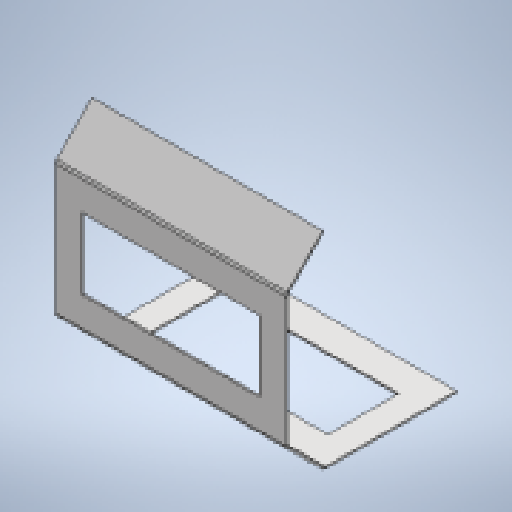
# Autodesk Inventor part: ANP 1454 BOTTOM DS box wall 1
Saved by Autodesk Inventor 2025 (Build 290162010, 162A)
## iProperties
Created: 2024-12-09
Part Number: ANP 1454 BOTTOM DS box wall 1
Material: Stainless Steel
Document SubType Name: Sheet Metal
Designer: user
Mass: 3269.02 g
Surface Area: 1007.63 cm^2
Volume: 408.627 cm^3
Density: 8 g/cm^3
Flat Pattern Width: 41.5348 cm
Flat Pattern Length: 26 cm
Flat Pattern Area: 1079.9 cm^2
Sheet Metal Rule: AISI304 2mm Die16
Sheet Metal Width: 415,348 mm
Sheet Metal Length: 260,000 mm
Sheet Metal Area: 107990,454 mm^2
Appearance: Default
Author: user
Autodesk Inventor part; units mm, degrees
ref_plane "YZ Plane" through (0, 0, 0) normal (1, 0, 0) x (0, 1, 0)
ref_plane "XZ Plane" through (0, 0, 0) normal (0, 1, 0) x (-1, 0, 0)
ref_plane "XY Plane" through (0, 0, 0) normal (0, 0, 1) x (1, 0, 0)
sketch "Sketch1" plane through (0, 0, 0) normal (0, 0, 1) x (1, 0, 0)
  line L0 (130, 75) -> (-130, 75)
  line L1 (-130, 75) -> (-130, -75)
  line L2 (-130, -75) -> (130, -75)
  line L3 (130, -75) -> (130, 75)
  line L4 (130, 75) -> (-130, -75) construction
  line L5 (-130, 75) -> (130, -75) construction
  line L6 (100, 40) -> (-100, 40)
  line L7 (-100, 40) -> (-100, -40)
  line L8 (-100, -40) -> (100, -40)
  line L9 (100, -40) -> (100, 40)
  line L10 (100, 40) -> (-100, -40) construction
  line L11 (-100, 40) -> (100, -40) construction
  point P0 (0, 0)
  point P1 (0, 0)
  point P2 (0, 0)
  point P3 (100, 0)
  point P4 (130, 0)
  dimension "d34" = 200
  dimension "d35" = 80
  dimension "d51" = 30
  dimension "d53" = 30
  dimension "d54" = 35
  dimension "d56" = 150
  measures "d34" distance of L7.end L8.end
  measures "d35" distance of L8.end L6.start
  measures "d51" distance between parallel lines of L9 L3
  measures "d53" distance between parallel lines of L1 L7
  measures "d54" distance between parallel lines of L8 L2
  measures "d56" distance of L0.start L2.end
extrude "Plate1" add sketch "Sketch1" along normal blind 2
sketch "Sketch6" plane through (130, -73.5858, 1.4142) normal (0, -0.7071068, -0.7071068) x (1, 0, 0)
  line L0 (-260, 0) -> (0, 0)
  line L1 (0, 0) -> (0, 60)
  line L2 (0, 60) -> (-260, 60)
  line L3 (-260, 60) -> (-260, 0)
  constraints: 6 end point, 1 horizontal, 1 perpendicular, 1 vertical
edge flange "Flange2" height 60 angle 45 thickness 2 bend radius 2.75 thickness toward (0, -0.7071068, -0.7071068) relief round relief width 2 relief depth 1 edges at (0, -75, 2) wall of the first edge with corners at (-130, -73.5858, 1.4142) (130, -73.5858, 1.4142) (130, -116.0122, 43.8406) (-130, -116.0122, 43.8406)
bend "Bend2"
corner "Corner2"
sketch "Sketch8" plane through (130, -115.4264, 42.4264) normal (0, -1, 0) x (1, 0, 0)
  line L0 (-260, 0) -> (0, 0)
  line L1 (0, 0) -> (0, 150)
  line L2 (0, 150) -> (-260, 150)
  line L3 (-260, 150) -> (-260, 0)
  constraints: 6 end point, 1 horizontal, 1 perpendicular, 1 vertical
edge flange "Flange3" height 150 angle 45 thickness 2 bend radius 2.75 thickness toward (0, -1, 0) relief round relief width 2 relief depth 1 edges at (0, -116.0122, 43.8406) wall of the first edge with corners at (-130, -115.4264, 42.4264) (130, -115.4264, 42.4264) (130, -115.4264, 192.4264) (-130, -115.4264, 192.4264)
bend "Bend3"
corner "Corner3"
sketch "Sketch9" plane through (130, -116.0122, 191.0122) normal (0, -0.7071068, 0.7071068) x (1, 0, 0)
  line L0 (-260, 0) -> (0, 0)
  line L1 (0, 0) -> (0, 58.6)
  line L2 (0, 58.6) -> (-260, 58.6)
  line L3 (-260, 58.6) -> (-260, 0)
  constraints: 6 end point, 1 horizontal, 1 perpendicular, 1 vertical
edge flange "Flange4" height 58.6 angle 45 thickness 2 bend radius 2.75 thickness toward (0, -0.7071068, 0.7071068) relief round relief width 2 relief depth 1 edges at (0, -115.4264, 192.4264) wall of the first edge with corners at (-130, -116.0122, 191.0122) (130, -116.0122, 191.0122) (130, -74.5757, 232.4487) (-130, -74.5757, 232.4487)
bend "Bend4"
corner "Corner4"
sketch "Sketch10" plane through (-130, -117.4264, 44.3939) normal (0, -1, 0) x (1, 0, 0)
  line L0 (260, 146.065) -> (0, 146.065) projected
  line L1 (0, 0) -> (0, 146.065) projected
  line L2 (0, 0) -> (260, 0) projected
  line L3 (260, 146.065) -> (260, 0) projected
  line L4 (30, 33.0325) -> (230, 33.0325)
  line L5 (230, 33.0325) -> (230, 113.0325)
  line L6 (230, 113.0325) -> (30, 113.0325)
  line L7 (30, 113.0325) -> (30, 33.0325)
  point P0 (130, -44.3939)
  point P1 (30, 73.0325)
  point P2 (0, 73.0325)
  dimension "d77" = 80
  dimension "d78" = 200
  dimension "d79" = 30
  constraints: 8 end point, 2 midpoint, 2 parallel, 1 horizontal, 1 horizontal alignment, 1 perpendicular
  measures "d77" distance of L6.end L4.start
  measures "d78" distance of L5.end L6.end
  measures "d79" distance between parallel lines of L7 L1
extrude "Cut3" cut sketch "Sketch10" against normal blind 2 contours L7 L6 L5 L4
sketch "Sketch11" plane through (0, 0, 0) normal (0, 0, -1) x (-1, 0, 0)
  line L0 (100, -40) -> (-100, -40) construction
  line L1 (-100, -40) -> (-100, 40) construction
  line L2 (-100, 40) -> (100, 40) construction
  line L3 (100, 40) -> (100, -40) construction
  circle A0 centre (0, -53) radius 2.75
  circle A1 centre (0, 53) radius 2.75
  line L4 (-100, 0) -> (100, 0) construction
  point P0 (0, 0)
  dimension "d82" = 106
  dimension "d83" = 5.5
  constraints: 2 centre point, 2 end point, 2 midpoint, 2 vertical alignment, 1 other
  measures "d82" distance of A1.centre A0.centre
  measures "d83" diameter of A0
extrude "Cut4" cut sketch "Sketch11" against normal blind 2
pattern_linear "Rectangular Pattern1" count 3 spacing 113 along (1, 0, 0) of "Cut4" first direction both ways yes
ref_plane "Work Plane1" through (0, -117.4264, 0) normal (0, 0.7071068, -0.7071068) x (1, 0, 0)
mirror "Mirror1" about plane through (0, -117.4264, 0) normal (0, 0.7071068, -0.7071068) of "Cut4", "Rectangular Pattern1"
equation "\"d34\" = MAIN_6_central_window_hight"
equation "\"d35\" = MAIN_7_central_window_width"
equation "\"d56\" = Wall_1_width"
equation "\"d77\" = MAIN_7_central_window_width"
equation "\"d78\" = MAIN_6_central_window_hight"
equation "\"d79\" = d53"
equation "\"d80\" = Thickness"
equation "\"d84\" = Thickness"
equation "\"d2\" = Thickness"
equation "\"d36\" = BendReliefWidth"
equation "\"d37\" = BendReliefDepth"
equation "\"d38\" = MinimumRemnant"
equation "\"d39\" = TransitionRadius"
equation "\"d40\" = Wall_2_width"
equation "\"d42\" = BendRadius"
equation "\"d43\" = CornerReliefSize"
equation "\"d44\" = GapSize"
equation "\"d45\" = JacobiRadiusSize"
equation "\"d57\" = BendReliefWidth"
equation "\"d58\" = BendReliefDepth"
equation "\"d59\" = MinimumRemnant"
equation "\"d60\" = TransitionRadius"
equation "\"d61\" = d56"
equation "\"d63\" = BendRadius"
equation "\"d64\" = CornerReliefSize"
equation "\"d65\" = GapSize"
equation "\"d66\" = JacobiRadiusSize"
equation "\"d67\" = BendReliefWidth"
equation "\"d68\" = BendReliefDepth"
equation "\"d69\" = MinimumRemnant"
equation "\"d70\" = TransitionRadius"
equation "\"d71\" = Wall_2_width - 0.7 * Thickness"
equation "\"d73\" = BendRadius"
equation "\"d74\" = CornerReliefSize"
equation "\"d75\" = GapSize"
equation "\"d76\" = JacobiRadiusSize"
equation "\"BendReliefWidth\" = Thickness"
equation "\"BendReliefDepth\" = 0.5 * Thickness"
equation "\"CornerReliefSize\" = 4 * Thickness"
equation "\"MinimumRemnant\" = 2 * Thickness"
equation "\"TransitionRadius\" = BendRadius"
equation "\"JacobiRadiusSize\" = BendRadius"
equation "\"GapSize\" = Thickness"
equation "\"MAIN_6_central_window_hight\" = 200"
equation "\"MAIN_7_central_window_width\" = 80"
equation "\"Wall_1_width\" = 150"
equation "\"Thickness\" = 2"
equation "\"Wall_2_width\" = 60"
equation "\"BendRadius\" = 2.75"
body "Solid1"
